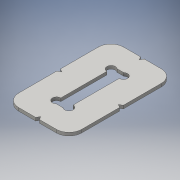
# Autodesk Inventor part: pcb-holder
Saved by Autodesk Inventor 2016 (Build 200138000, 138)
## iProperties
Created: 2022-06-29
Part Number: pcb-holder
Material: Generic
Document SubType Name: Modeling
Designer: Teemu S.
Density: 1 g/cm^3
Appearance: Default
Author: Teemu S.
Autodesk Inventor part; units mm, degrees
ref_plane "YZ Plane" through (0, 0, 0) normal (1, 0, 0) x (0, 1, 0)
ref_plane "XZ Plane" through (0, 0, 0) normal (0, 1, 0) x (-1, 0, 0)
ref_plane "XY Plane" through (0, 0, 0) normal (0, 0, 1) x (1, 0, 0)
sketch "Sketch2" plane through (0, 0, 0) normal (0, 0, 1) x (1, 0, 0)
  line L0 (0, 0) -> (144, 0) construction
  line L1 (144, 0) -> (144, -204) construction
  line L2 (144, -204) -> (0, -204) construction
  line L3 (0, -204) -> (0, 0) construction
  circle A0 centre (135, -27) radius 3 construction
  circle A1 centre (122, -9) radius 3 construction
  circle A2 centre (135, -177) radius 3 construction
  circle A3 centre (122, -195) radius 3 construction
  circle A4 centre (22, -195) radius 3 construction
  circle A5 centre (9, -177) radius 3 construction
  circle A6 centre (9, -27) radius 3 construction
  circle A7 centre (22, -9) radius 3 construction
  line L4 (12, -12) -> (132, -12) construction
  line L5 (132, -12) -> (132, -192) construction
  line L6 (132, -192) -> (12, -192) construction
  line L7 (12, -192) -> (12, -12) construction
  circle A8 centre (22, -9) radius 2.925
  circle A9 centre (9, -27) radius 2.925
  circle A10 centre (122, -9) radius 2.925
  circle A11 centre (135, -27) radius 2.925
  circle A12 centre (135, -177) radius 2.925
  circle A13 centre (122, -195) radius 2.925
  circle A14 centre (22, -195) radius 2.925
  circle A15 centre (9, -177) radius 2.925
  line L8 (122, -9) -> (135, -9) construction
  line L9 (135, -9) -> (135, -27) construction
  line L10 (126, -27) -> (126, -18)
  line L11 (126, -18) -> (122, -18)
  line L12 (144, -27) -> (144, 0)
  line L13 (144, 0) -> (122, 0)
  line L14 (122, -195) -> (135, -195) construction
  line L15 (135, -195) -> (135, -177) construction
  line L16 (126, -177) -> (126, -186)
  line L17 (126, -186) -> (122, -186)
  line L18 (144, -177) -> (144, -204)
  line L19 (144, -204) -> (122, -204)
  line L20 (126, -27) -> (126, -177)
  line L21 (144, -177) -> (144, -27)
  line L22 (122, -9) -> (113, -9) construction
  line L23 (122, 0) -> (113, 0)
  line L24 (122, -18) -> (113, -18)
  line L25 (113, -18) -> (113, 0)
  line L26 (122, -195) -> (113, -195) construction
  line L27 (122, -204) -> (113, -204)
  line L28 (122, -186) -> (113, -186)
  line L29 (113, -186) -> (113, -204)
  line L30 (75.025, -87) -> (68.975, -87) construction
  line L31 (68.975, -87) -> (68.975, -117) construction
  line L32 (68.975, -117) -> (75.025, -117) construction
  line L33 (75.025, -117) -> (75.025, -87) construction
  line L34 (74.935, -87.5) -> (73.6121, -87.5)
  line L35 (69.065, -87.5) -> (69.065, -91)
  line L36 (69.065, -116.5) -> (70.3879, -116.5)
  line L37 (74.935, -116.5) -> (74.935, -113)
  arc A16 (73.6121, -116.5) -> (74.935, -113) centre (74.935, -115) ccw
  arc A17 (69.065, -113) -> (70.3879, -116.5) centre (69.065, -115) ccw
  arc A18 (74.935, -91) -> (73.6121, -87.5) centre (74.935, -89) ccw
  arc A19 (70.3879, -87.5) -> (69.065, -91) centre (69.065, -89) ccw
  line L38 (69.065, -91) -> (69.065, -113)
  line L39 (70.3879, -87.5) -> (69.065, -87.5)
  line L40 (73.6121, -87.5) -> (70.3879, -87.5)
  line L41 (74.935, -91) -> (74.935, -87.5)
  line L42 (74.935, -113) -> (74.935, -91)
  line L43 (70.3879, -116.5) -> (73.6121, -116.5)
  line L44 (73.6121, -116.5) -> (74.935, -116.5)
  line L45 (69.065, -113) -> (69.065, -116.5)
  arc A20 (69.065, -91) -> (70.3879, -87.5) centre (69.065, -89) ccw
  arc A21 (73.6121, -87.5) -> (74.935, -91) centre (74.935, -89) ccw
  arc A22 (74.935, -113) -> (73.6121, -116.5) centre (74.935, -115) ccw
  arc A23 (70.3879, -116.5) -> (69.065, -113) centre (69.065, -115) ccw
  line L46 (57, -127) -> (87, -127)
  line L47 (87, -127) -> (87, -77)
  line L48 (87, -77) -> (57, -77)
  line L49 (57, -77) -> (57, -127)
  point P0 (132, -102)
  point P1 (144, -102)
  point P2 (72, -12)
  point P3 (72, 0)
  point P4 (72, -87)
  point P5 (75.025, -102)
  point P6 (74.935, -102)
  point P7 (72, -87.5)
  point P8 (74.935, -102)
  point P9 (72, -87.5)
  point P10 (72, -77)
  point P11 (87, -102)
  dimension "d0" = 144
  dimension "d1" = 204
  dimension "d2" = 6
  dimension "d3" = 6
  dimension "d4" = 6
  dimension "d5" = 6
  dimension "d6" = 6
  dimension "d7" = 6
  dimension "d8" = 6
  dimension "d9" = 6
  dimension "d10" = 120
  dimension "d11" = 180
  dimension "d12" = 15
  dimension "d13" = 10
  dimension "d14" = 10
  dimension "d15" = 15
  dimension "d16" = 15
  dimension "d17" = 10
  dimension "d18" = 10
  dimension "d19" = 15
  dimension "d20" = 0.075
  dimension "d21" = 0.075
  dimension "d22" = 0.075
  dimension "d23" = 0.075
  dimension "d24" = 0.075
  dimension "d25" = 0.075
  dimension "d26" = 0.075
  dimension "d27" = 0.075
  dimension "d28" = 9
  dimension "d29" = 9
  dimension "d30" = 9
  dimension "d31" = 9
  dimension "d32" = 9
  dimension "d33" = 9
  dimension "d34" = 6.05
  dimension "d35" = 30
  dimension "d36" = 29
  dimension "d37" = 5.87
  dimension "d38" = 4
  dimension "d39" = 1.5
  dimension "d40" = 4
  dimension "d41" = 1.5
  dimension "d42" = 1.5
  dimension "d43" = 1.5
  dimension "d44" = 4
  dimension "d45" = 4
  dimension "d54" = 30
  dimension "d55" = 50
  constraints: 100 end point, 26 parallel, 24 centre point, 21 perpendicular, 16 point on circle, 13 horizontal, 12 midpoint, 9 point on line, 8 coincident, 8 tangent, 5 horizontal alignment, 5 vertical alignment, 4 other
  measures "d0" distance of L1.end L2.end
  measures "d1" distance of L0.end L1.end
  measures "d2" diameter of A0
  measures "d3" diameter of A1
  measures "d4" diameter of A2
  measures "d5" diameter of A3
  measures "d6" diameter of A4
  measures "d7" diameter of A5
  measures "d8" diameter of A6
  measures "d9" diameter of A7
  measures "d10" distance of L5.end L6.end
  measures "d11" distance of L4.end L5.end
  measures "d12" vertical distance of A0.centre L4.end
  measures "d13" horizontal distance of L4.end A1.centre
  measures "d14" horizontal distance of L4.start A7.centre
  measures "d15" vertical distance of L4.start A6.centre
  measures "d16" vertical distance of L6.end A5.centre
  measures "d17" horizontal distance of A4.centre L6.end
  measures "d18" horizontal distance of L5.end A3.centre
  measures "d19" vertical distance of L5.end A2.centre
  measures "d20" radial gap between concentric circles of A5 A15
  measures "d21" radial gap between concentric circles of A4 A14
  measures "d22" radial gap between concentric circles of A6 A9
  measures "d23" radial gap between concentric circles of A7 A8
  measures "d24" radial gap between concentric circles of A1 A10
  measures "d25" radial gap between concentric circles of A0 A11
  measures "d26" radial gap between concentric circles of A2 A12
  measures "d27" radial gap between concentric circles of A3 A13
  measures "d28" distance between parallel lines of L9 L10
  measures "d29" distance between parallel lines of L9 L12
  measures "d30" distance between parallel lines of L15 L16
  measures "d31" distance between parallel lines of L15 L18
  measures "d32" distance of L8.start L22.end
  measures "d33" distance of L14.start L26.end
  measures "d34" distance of L32.end L31.end
  measures "d35" distance of L30.end L31.end
  measures "d36" distance of L37.start L34.start
  measures "d37" distance of L34.start L35.start
  measures "d38" diameter of A16
  measures "d39" distance of A16.centre L37.start
  measures "d40" diameter of A17
  measures "d41" distance of L36.start A17.centre
  measures "d42" distance of L34.start A18.centre
  measures "d43" distance of L35.start A19.centre
  measures "d44" diameter of A18
  measures "d45" diameter of A19
  measures "d54" distance of L47.end L48.end
  measures "d55" distance of L48.end L46.start
extrude "Extrusion1" add sketch "Sketch2" along normal blind 1.5 contours L49 L48 L47 L46
sketch "Sketch3" plane through (0, 0, 1.5) normal (0, 0, 1) x (1, 0, 0)
  line L0 (87, -77) -> (57, -77) construction
  line L1 (72, -77) -> (72, -78.5) construction
  line L2 (57, -127) -> (87, -127) construction
  line L3 (72, -127) -> (72, -125.5) construction
  line L4 (57, -77) -> (57, -127) construction
  line L5 (57, -102) -> (58.5, -102) construction
  line L6 (87, -127) -> (87, -77) construction
  line L7 (87, -102) -> (85.5, -102) construction
  line L8 (72, -78.5) -> (72.866, -77)
  line L9 (72, -78.5) -> (73.7321, -78.5) construction
  line L10 (72, -78.5) -> (71.134, -77)
  line L11 (71.134, -77) -> (72.866, -77)
  line L12 (72, -125.5) -> (72.866, -127)
  line L13 (72, -125.5) -> (71.134, -127)
  line L14 (72.866, -127) -> (71.134, -127)
  line L15 (58.5, -102) -> (57, -101.134)
  line L16 (57, -102.866) -> (58.5, -102)
  line L17 (57, -101.134) -> (57, -102.866)
  line L18 (85.5, -102) -> (87, -101.134)
  line L19 (85.5, -102) -> (87, -102.866)
  line L20 (87, -101.134) -> (87, -102.866)
  point P0 (0, 0)
  dimension "d59" = 1.5
  dimension "d60" = 1.5
  dimension "d61" = 1.5
  dimension "d62" = 1.5
  dimension "d63" = 60
  dimension "d64" = 60
  dimension "d65" = 60
  dimension "d66" = 60
  dimension "d67" = 60
  constraints: 34 end point, 8 point on line, 4 midpoint, 3 collinear, 3 horizontal, 2 parallel, 2 vertical, 1 equal length, 3 other
  measures "d59" distance of L1.start L1.end
  measures "d60" distance of L3.start L3.end
  measures "d61" distance of L5.start L5.end
  measures "d62" distance of L7.start L7.end
  measures "d63" angle of L9 L8
  measures "d64" angle of L8 L10
  measures "d65" angle of L12 L13
  measures "d66" angle of L18 L19
  measures "d67" angle of L15 L16
extrude "Extrusion2" cut sketch "Sketch3" against normal blind 1.5
fillet "Fillet1" radius 6 4 edges at (57, -127, 0.75) (87, -127, 0.75) (87, -77, 0.75) (57, -77, 0.75)
equation "\"d0\" = d46"
equation "\"d1\" = d47"
equation "\"d2\" = d48"
equation "\"d3\" = d48"
equation "\"d4\" = d48"
equation "\"d5\" = d48"
equation "\"d6\" = d48"
equation "\"d7\" = d48"
equation "\"d8\" = d48"
equation "\"d9\" = d48"
equation "\"d10\" = d49"
equation "\"d11\" = d50"
equation "\"d12\" = d51"
equation "\"d13\" = d52"
equation "\"d14\" = d52"
equation "\"d15\" = d51"
equation "\"d16\" = d51"
equation "\"d17\" = d52"
equation "\"d18\" = d52"
equation "\"d19\" = d51"
equation "\"d20\" = d53"
equation "\"d21\" = d53"
equation "\"d22\" = d53"
equation "\"d23\" = d53"
equation "\"d24\" = d53"
equation "\"d25\" = d53"
equation "\"d26\" = d53"
equation "\"d27\" = d53"
equation "\"d28\" = 1.5 * d48"
equation "\"d29\" = 1.5 * d48"
equation "\"d30\" = 1.5 * d48"
equation "\"d31\" = 1.5 * d48"
equation "\"d32\" = 1.5 * d48"
equation "\"d33\" = 1.5 * d48"
equation "\"d40\" = d38"
equation "\"d41\" = d39"
equation "\"d42\" = d39"
equation "\"d43\" = d42"
equation "\"d44\" = d38"
equation "\"d45\" = d38"
equation "\"d60\" = d59"
equation "\"d61\" = d59"
equation "\"d62\" = d59"
equation "\"d46\" = 144"
equation "\"d47\" = 204"
equation "\"d48\" = 6"
equation "\"d49\" = 120"
equation "\"d50\" = 180"
equation "\"d51\" = 15"
equation "\"d52\" = 10"
equation "\"d53\" = 0.075"
body "Solid1"
